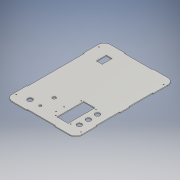
# Autodesk Inventor part: Panel
Saved by Autodesk Inventor 2016 (Build 200138000, 138)
## iProperties
Created: 2016-03-26
Part Number: Panel
Material: Acetal Resin, Black
Document SubType Name: Sheet Metal
Designer: agmle
Density: 1.425 g/cm^3
Sheet Metal Rule: Default
Appearance: Smooth - White
Author: agmle
Autodesk Inventor part; units mm, degrees
ref_plane "YZ Plane" through (0, 0, 0) normal (1, 0, 0) x (0, 1, 0)
ref_plane "XZ Plane" through (0, 0, 0) normal (0, 1, 0) x (-1, 0, 0)
ref_plane "Work Plane1" through (300.7927, 694.1728, 0) normal (0, 0, 1) x (1, -0.0015, 0)
sketch "Sketch1" plane through (300.7927, 694.1728, 0) normal (0, 0, 1) x (1, -0.0015, 0)
  line L0 (11.0652, -476.8683) -> (-44.7258, -476.9512) construction
  arc A0 (11.0652, -476.8683) -> (35.1594, -452.7025) centre (11.0294, -452.7384) ccw construction
  line L1 (35.0759, -396.5178) -> (35.1594, -452.7025) construction
  line L2 (32.2566, -396.522) -> (35.0759, -396.5178) construction
  line L3 (32.109, -297.1065) -> (32.2566, -396.522) construction
  line L4 (34.9284, -297.1023) -> (32.109, -297.1065) construction
  line L5 (34.845, -240.9176) -> (34.9284, -297.1023) construction
  arc A1 (34.845, -240.9176) -> (10.6792, -216.8234) centre (10.715, -240.9534) ccw construction
  line L6 (-45.1119, -216.9062) -> (10.6792, -216.8234) construction
  line L7 (-45.1077, -219.7256) -> (-45.1119, -216.9062) construction
  line L8 (-129.6388, -219.8511) -> (-45.1077, -219.7256) construction
  line L9 (-129.643, -217.0317) -> (-129.6388, -219.8511) construction
  line L10 (-166.4983, -217.0864) -> (-129.643, -217.0317) construction
  line L11 (-166.4942, -219.9058) -> (-166.4983, -217.0864) construction
  line L12 (-251.0253, -220.0313) -> (-166.4942, -219.9058) construction
  line L13 (-251.0295, -217.2119) -> (-251.0253, -220.0313) construction
  line L14 (-306.8205, -217.2948) -> (-251.0295, -217.2119) construction
  arc A2 (-306.8205, -217.2948) -> (-330.9146, -241.4606) centre (-306.7847, -241.4247) ccw construction
  line L15 (-330.8312, -297.6453) -> (-330.9146, -241.4606) construction
  line L16 (-328.0118, -297.6411) -> (-330.8312, -297.6453) construction
  line L17 (-327.8643, -397.0566) -> (-328.0118, -297.6411) construction
  line L18 (-330.6836, -397.0608) -> (-327.8643, -397.0566) construction
  line L19 (-330.6002, -453.2455) -> (-330.6836, -397.0608) construction
  arc A3 (-330.6002, -453.2455) -> (-306.4344, -477.3397) centre (-306.4703, -453.2097) ccw construction
  line L20 (-250.6434, -477.2569) -> (-306.4344, -477.3397) construction
  line L21 (-250.6476, -474.4375) -> (-250.6434, -477.2569) construction
  line L22 (-44.73, -474.1318) -> (-250.6476, -474.4375) construction
  line L23 (-44.7258, -476.9512) -> (-44.73, -474.1318) construction
  circle A4 centre (4.6999, -466.5639) radius 1.0795 construction
  circle A5 centre (-300.0998, -467.0164) radius 1.0795 construction
  circle A6 centre (-300.4552, -227.5992) radius 1.0795 construction
  circle A7 centre (4.3445, -227.1467) radius 1.0795 construction
  line L24 (-251.9195, -473.1693) -> (-251.9153, -475.9887)
  line L25 (-251.9153, -475.9887) -> (-306.4363, -476.0697)
  arc A8 (-329.3302, -453.2436) -> (-306.4363, -476.0697) centre (-306.4703, -453.2097) ccw
  line L26 (-329.3302, -453.2436) -> (-329.4118, -398.3289)
  line L27 (-329.4118, -398.3289) -> (-326.5924, -398.3247)
  line L28 (-326.5924, -398.3247) -> (-326.7437, -296.3692)
  line L29 (-326.7437, -296.3692) -> (-329.5631, -296.3734)
  line L30 (-329.5631, -296.3734) -> (-329.6446, -241.4587)
  arc A9 (-306.8186, -218.5648) -> (-329.6446, -241.4587) centre (-306.7847, -241.4247) ccw
  line L31 (-306.8186, -218.5648) -> (-252.2976, -218.4838)
  line L32 (-252.2976, -218.4838) -> (-252.2934, -221.3032)
  line L33 (-252.2934, -221.3032) -> (-165.2223, -221.174)
  line L34 (-165.2223, -221.174) -> (-165.2265, -218.3546)
  line L35 (-165.2265, -218.3546) -> (-130.9111, -218.3036)
  line L36 (-130.9111, -218.3036) -> (-130.9069, -221.123)
  line L37 (-130.9069, -221.123) -> (-43.8358, -220.9938)
  line L38 (-43.8358, -220.9938) -> (-43.84, -218.1744)
  line L39 (-43.84, -218.1744) -> (10.681, -218.0934)
  arc A10 (33.575, -240.9195) -> (10.681, -218.0934) centre (10.715, -240.9534) ccw
  line L40 (33.575, -240.9195) -> (33.6565, -295.8342)
  line L41 (33.6565, -295.8342) -> (30.8371, -295.8384)
  line L42 (30.8371, -295.8384) -> (30.9884, -397.7939)
  line L43 (30.9884, -397.7939) -> (33.8078, -397.7897)
  line L44 (33.8078, -397.7897) -> (33.8894, -452.7044)
  arc A11 (11.0633, -475.5983) -> (33.8894, -452.7044) centre (11.0294, -452.7384) ccw
  line L45 (11.0633, -475.5983) -> (-43.4577, -475.6793)
  line L46 (-43.4577, -475.6793) -> (-43.4619, -472.8599)
  line L47 (-43.4619, -472.8599) -> (-251.9195, -473.1693)
  dimension "d32" = 1.27
  measures "d32" distance between parallel lines of L22 L47
extrude "Plate1" add sketch "Sketch1" along normal blind 3.048
sketch "Sketch3" plane through (300.7927, 694.1728, 0) normal (0, 0, -1) x (-1, 0.0015, 0)
  circle A0 centre (300.2757, -466.9836) radius 1.0795 construction
  circle A1 centre (-4.5243, -466.9836) radius 1.0795 construction
  circle A2 centre (-4.5243, -227.5661) radius 1.0795 construction
  circle A3 centre (300.2757, -227.5661) radius 1.0795 construction
  line L0 (-4.5243, -227.5661) -> (300.2757, -227.5661) construction
  line L1 (300.2757, -227.5661) -> (300.2757, -466.9836) construction
  line L2 (300.2757, -466.9836) -> (-4.5243, -466.9836) construction
  line L3 (-4.5243, -466.9836) -> (-4.5243, -227.5661) construction
  line L4 (326.5924, -398.3247) -> (326.7437, -296.3692) construction
  line L5 (326.668, -347.347) -> (300.2757, -347.2749) construction
  line L6 (43.4619, -472.8599) -> (251.9195, -473.1693) construction
  line L7 (165.2265, -218.3546) -> (130.9111, -218.3036) construction
  line L8 (-4.5243, -347.2749) -> (-30.9128, -346.8161) construction
  line L9 (-30.8371, -295.8384) -> (-30.9884, -397.7939) construction
  point P0 (152.4, -347.3112)
  dimension "d2" = 304.8
  dimension "d3" = 239.4175
  constraints: 12 end point, 6 coincident, 4 midpoint, 2 parallel, 1 equal length, 1 horizontal, 1 perpendicular
  measures "d2" distance of L0.start L0.end
  measures "d3" distance of L0.end L1.end
hole "Mounting_Holes" at (0.1795, 467.0527, 0) at (-0.1759, 227.6355, 0) at (304.6238, 227.183, 0) at (304.9792, 466.6002, 0) direction (0, 0, 1) diameter 3.2766 end through all clearance for "Flat Head Machine Screw (82)" size "#4" standard "Ansi Unified Screw Threads"
sketch "Sketch4" plane through (300.7927, 694.1728, 0) normal (0, 0, -1) x (-1, 0.0015, 0)
  circle A0 centre (4.2521, -424.821) radius 10.541 construction
  line L0 (-33.575, -240.9195) -> (-33.6565, -295.8342) projected
  line L1 (43.84, -218.1744) -> (-10.681, -218.0934) projected
  line L2 (-11.0633, -475.5983) -> (43.4577, -475.6793) projected
  dimension "d11" = 21.082
  dimension "d33" = 38.1
  dimension "d86" = 50.8
  constraints: 1 centre point, 1 coincident
  measures "d11" diameter of A0
  measures "d33" distance from line of L0 point (4.252, -424.821)
  measures "d86" distance from line of L2 point (4.252, -424.821)
hole "Power_Connector" at (295.91, 269.3586, 0) direction (0, 0, 1) diameter 17.4752 end through all thread size "1/2" designation "1/2 - 14 NPT" standard "NPT for PVC Pipe and Fitting"
sketch "Sketch7" plane through (300.7927, 694.1728, 3.048) normal (0, 0, 1) x (1, -0.0015, 0)
  line L0 (0.8093, -320.4599) -> (-98.1907, -320.4599)
  line L1 (-98.1907, -320.4599) -> (-98.1907, -278.9599)
  line L2 (-98.1907, -278.9599) -> (0.8093, -278.9599)
  line L3 (0.8093, -278.9599) -> (0.8093, -320.4599)
  line L4 (-165.2265, -218.3546) -> (-130.9111, -218.3036) construction
  line L5 (-43.4619, -472.8599) -> (-251.9195, -473.1693) construction
  line L6 (-43.4619, -472.8599) -> (-251.9195, -473.1693) construction
  line L7 (-147.6907, -473.0146) -> (-147.7272, -448.3951) construction
  point P0 (-299.7619, -694.6186)
  dimension "d40" = 99
  dimension "d41" = 41.5
  dimension "d80" = 152.4
  dimension "d81" = 49.5
  constraints: 10 end point, 2 parallel, 2 perpendicular, 1 horizontal, 1 midpoint
  measures "d40" distance of L0.start L0.end
  measures "d41" distance of L2.end L0.start
  measures "d80" distance from line of L5.start L0
  measures "d81" distance from line of L7.start L1
extrude "LCD_Cutout" cut sketch "Sketch7" against normal through all
sketch "Sketch8" plane through (300.7927, 694.1728, 3.048) normal (0, 0, 1) x (1, -0.0015, 0)
  line L0 (-1.6907, -327.2099) -> (-95.6907, -327.2099) construction
  line L1 (-95.6907, -327.2099) -> (-95.6907, -272.2099) construction
  line L2 (-95.6907, -272.2099) -> (-1.6907, -272.2099) construction
  line L3 (-1.6907, -272.2099) -> (-1.6907, -327.2099) construction
  line L4 (-48.6907, -327.2099) -> (-48.6907, -320.4599) construction
  line L5 (0.8093, -320.4599) -> (-98.1907, -320.4599) construction
  line L6 (-98.1907, -278.9599) -> (0.8093, -278.9599) construction
  line L7 (-48.6907, -278.9599) -> (-48.6907, -272.2099) construction
  point P0 (-299.7619, -694.6186)
  dimension "d45" = 94
  dimension "d46" = 55
  constraints: 12 end point, 4 coincident, 4 midpoint, 2 collinear, 2 parallel, 1 horizontal, 1 perpendicular
  measures "d45" distance of L0.start L0.end
  measures "d46" distance of L2.end L0.start
hole "LCD_Holes" at (298.6163, 366.9658, 3.048) at (204.6164, 367.1053, 3.048) at (204.698, 422.1053, 3.048) at (298.6979, 421.9657, 3.048) direction (0, 0, -1) diameter 3.2766 end through all clearance for "Socket Head Cap Screw" size "#4" standard "Ansi Unified Screw Threads"
sketch "Sketch9" plane through (300.7927, 694.1728, 3.048) normal (0, 0, 1) x (1, -0.0015, 0)
  circle A0 centre (-4.2521, -424.821) radius 9.0607 projected
  line L0 (30.8371, -295.8384) -> (30.9884, -397.7939) projected
  point P0 (-299.7619, -694.6186)
  point P1 (-55.0521, -386.721)
  dimension "d84" = 50.8
  dimension "d85" = 38.1
  measures "d84" horizontal distance of point (-55.052, -386.721) A0.centre
  measures "d85" vertical distance of A0.centre point (-55.052, -386.721)
hole "Pickle_Switch" at (245.1666, 307.5339, 3.048) direction (0, 0, -1) diameter 12 end through all
sketch "Sketch10" plane through (300.7927, 694.1728, 3.048) normal (0, 0, 1) x (1, -0.0015, 0)
  line L0 (-15.1907, -253.5599) -> (-82.1907, -253.5599) construction
  line L1 (-98.1907, -278.9599) -> (0.8093, -278.9599) construction
  line L2 (-48.6907, -278.9599) -> (-48.6907, -253.5599) construction
  line L3 (0.8093, -278.9599) -> (0.8093, -320.4599) construction
  point P0 (-299.7619, -694.6186)
  dimension "d62" = 16
  dimension "d63" = 25.4
  constraints: 4 end point, 2 midpoint, 1 coincident, 1 parallel, 1 perpendicular
  measures "d62" distance from line of L3 L0.start
  measures "d63" distance of L2.start L2.end
hole "Pushbuttons" at (285.2256, 440.6357, 3.048) at (251.7257, 440.6855, 3.048) at (218.2257, 440.7352, 3.048) direction (0, 0, -1) diameter 17.5006 end through all clearance for "Hex Head Cap Screw ISO 24017" size "M16" standard "ISO"
sketch "Sketch11" plane through (300.7927, 694.1728, 3.048) normal (0, 0, 1) x (1, -0.0015, 0)
  circle A0 centre (-4.2521, -424.821) radius 9.0607 construction
  circle A1 centre (-55.0521, -386.721) radius 6 construction
  line L0 (-4.2521, -424.821) -> (-4.2521, -386.721) construction
  point P0 (-299.7619, -694.6186)
  dimension "d71" = 38.1
  constraints: 2 end point, 1 vertical
  measures "d71" distance of L0.start L0.end
hole "Air_Coupler" at (295.9666, 307.4585, 3.048) direction (0, 0, -1) diameter 8.89 depth 3.048 tip angle 118
sketch "Sketch12" plane through (300.7927, 694.1728, 3.048) normal (0, 0, 1) x (1, -0.0015, 0)
  line L0 (-250.9997, -426.9053) -> (-287.5757, -426.9053)
  line L1 (-287.5757, -426.9053) -> (-287.5757, -405.3661)
  line L2 (-287.5757, -405.3661) -> (-250.9997, -405.3661)
  line L3 (-250.9997, -405.3661) -> (-250.9997, -426.9053)
  circle A0 centre (-300.2757, -227.5661) radius 1.6383 construction
  point P0 (-299.7619, -694.6186)
  dimension "d87" = 36.576
  dimension "d88" = 21.5392
  dimension "d89" = 177.8
  dimension "d90" = 12.7
  constraints: 8 end point, 2 parallel, 1 horizontal, 1 perpendicular
  measures "d87" distance of L1.end L2.end
  measures "d88" distance of L0.end L1.end
  measures "d89" distance from line of A0.centre L2
  measures "d90" distance from line of A0.centre L1
extrude "Powerpole_Cutout" cut sketch "Sketch12" against normal blind 3.048
sketch "Sketch13" plane through (300.7927, 694.1728, 3.048) normal (0, 0, 1) x (1, -0.0015, 0)
  line L0 (-15.3261, -339.5099) -> (-44.6761, -339.5099) construction
  line L1 (30.8371, -295.8384) -> (30.9884, -397.7939) construction
  line L2 (0.8093, -320.4599) -> (-98.1907, -320.4599) construction
  point P0 (-299.7619, -694.6186)
  dimension "d93" = 46.228
  dimension "d94" = 29.35
  dimension "d95" = 19.05
  constraints: 2 coincident, 2 end point, 1 horizontal
  measures "d93" distance from line of L1 L0.start
  measures "d94" distance of L0.start L0.end
  measures "d95" distance between parallel lines of L2 L0
hole "Fan Bracket" at (284.9626, 354.686, 3.048) at (255.6126, 354.7296, 3.048) direction (0, 0, -1) diameter 3.2766 end through all clearance for "Socket Head Cap Screw" size "#4" standard "Ansi Unified Screw Threads"
equation "\"d9\" = Thickness"
equation "\"d43\" = Thickness"
equation "\"d45\" = LCD_PCB_Horizontal_Hole_Spacing"
equation "\"d46\" = LCD_PCB_Vertical_Hole_Spacing"
equation "\"d47\" = LCD_Cover_Hole_Diameter"
equation "\"d60\" = Thickness"
equation "\"d69\" = Thickness"
equation "\"d77\" = Thickness"
equation "\"d91\" = Thickness"
equation "\"d94\" = Bracket_Hole_Spacing"
equation "\"d101\" = Thickness"
equation "\"d81\" = 0.5 * d40"
equation "\"BendRadius\" = Thickness"
equation "\"BendReliefWidth\" = Thickness"
equation "\"BendReliefDepth\" = 0.5 * Thickness"
equation "\"CornerReliefSize\" = 4 * Thickness"
equation "\"MinimumRemnant\" = 2 * Thickness"
equation "\"TransitionRadius\" = BendRadius"
equation "\"JacobiRadiusSize\" = BendRadius"
equation "\"GapSize\" = Thickness"
equation "\"d1\" = BendRadius"
equation "\"Thickness\" = 3.048"
equation "\"LCD_PCB_Horizontal_Hole_Spacing\" = 94"
equation "\"LCD_PCB_Vertical_Hole_Spacing\" = 55"
equation "\"LCD_Cover_Hole_Diameter\" = 3.2766"
equation "\"Bracket_Hole_Spacing\" = 29.35"
body "Solid1"
